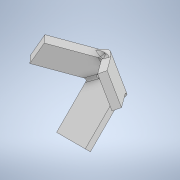
# Autodesk Inventor part: arm_holder_1
Saved by Autodesk Inventor 2020 (Build 240168000, 168)
## iProperties
Created: 2020-01-19
Part Number: arm_holder_1
Material: Generic
Document SubType Name: Modeling
Designer: psrobotics
Density: 1 g/cm^3
Appearance: Default
Author: psrobotics
Autodesk Inventor part; units mm, degrees
ref_plane "YZ Plane" through (0, 0, 0) normal (1, 0, 0) x (0, 1, 0)
ref_plane "XZ Plane" through (0, 0, 0) normal (0, 1, 0) x (-1, 0, 0)
ref_plane "XY Plane" through (0, 0, 0) normal (0, 0, 1) x (1, 0, 0)
sketch "Sketch1" plane through (0, 0, 0) normal (0, 0, 1) x (1, 0, 0)
  line L0 (0, 0) -> (20, 0)
  line L1 (20, 0) -> (10, 17.3205)
  line L2 (10, 17.3205) -> (0, 0)
  line L3 (10, 17.3205) -> (14.3301, 19.8205)
  line L4 (14.3301, 19.8205) -> (24.3301, 2.5)
  line L5 (24.3301, 2.5) -> (20, 0)
  line L6 (20, 0) -> (0, 0)
  line L7 (0, 0) -> (0, -5)
  line L8 (0, -5) -> (20, -5)
  line L9 (20, -5) -> (20, 0)
  line L10 (10, 17.3205) -> (5.6699, 19.8205)
  line L11 (5.6699, 19.8205) -> (-4.3301, 2.5)
  line L12 (-4.3301, 2.5) -> (0, 0)
  line L13 (5.6699, 19.8205) -> (14.3301, 19.8205)
  line L14 (20, -5) -> (24.3301, 2.5)
  line L15 (0, -5) -> (-4.3301, 2.5)
  dimension "d0" = 20
  dimension "d1" = 20
  dimension "d2" = 60
  dimension "d3" = 5
  dimension "d4" = 20
  dimension "d5" = 20
  dimension "d6" = 5
  dimension "d7" = 5
  dimension "d8" = 20
  dimension "d9" = 5
  constraints: 32 end point, 4 perpendicular, 2 horizontal, 2 parallel
  measures "d0" distance of L0.start L0.end
  measures "d1" distance of L0.end L1.end
  measures "d2" angle of L1 L0
  measures "d3" distance of L1.end L3.end
  measures "d4" distance of L3.end L4.end
  measures "d5" distance of L8.end L7.end
  measures "d6" distance of L7.end L6.end
  measures "d7" distance of L1.end L10.end
  measures "d8" distance of L10.end L11.end
  measures "d9" distance of L0.start L11.end
extrude "Extrusion1" add sketch "Sketch1" along normal blind 3 contours L12 L11 L10 L2 | L0 L9 L8 L7 | L7 L15 L12 | L1 L3 L4 L5 | L5 L14 L9 | L10 L13 L3
sketch "Sketch2" plane through (0, -5, 0) normal (0, -1, 0) x (1, 0, 0)
  line L0 (0, 0) -> (20, 0) projected
  line L1 (20, 0) -> (20, 3) projected
  line L2 (0, 3) -> (20, 3) projected
  line L3 (0, 0) -> (0, 3) projected
  line L4 (20, 3) -> (0, 3)
  line L5 (0, 3) -> (0, 23)
  line L6 (0, 23) -> (20, 23)
  line L7 (20, 23) -> (20, 3)
  dimension "d12" = 20
  dimension "d13" = 20
  constraints: 8 end point, 2 parallel, 1 horizontal, 1 perpendicular
  measures "d12" distance of L5.end L6.end
  measures "d13" distance of L4.end L5.end
extrude "Extrusion2" add sketch "Sketch2" along normal blind 20 contours L5 L6 L7 L2
sketch "Sketch3" plane through (0, -5, 3) normal (-1, 0, 0) x (0, 0, 1)
  line L0 (20, 0) -> (0, 0) projected
  line L1 (0, 0) -> (0, -20) projected
  line L2 (20, -20) -> (0, -20) projected
  line L3 (20, 0) -> (20, -20) projected
  line L4 (0, 0) -> (0, 7.5) projected
  line L5 (0, -20) -> (20, -20) projected
  line L6 (0, 0) -> (20, -20)
  point P0 (-3, 5)
  constraints: 2 end point
extrude "Extrusion3" cut sketch "Sketch3" against normal blind 20 contours L6 L2 L1
sketch "Sketch4" plane through (0, -5, 3) normal (-1, 0, 0) x (0, 0, 1)
  line L0 (0, 0) -> (20, -20) projected
  line L1 (20, 0) -> (20, -20) projected
  line L2 (20, 0) -> (0, 0) projected
  line L3 (0, 7.5) -> (0, 0) projected
  line L4 (20, -20) -> (23.5355, -16.4645)
  line L5 (0, 0) -> (20, -20) projected
  line L6 (23.5355, -16.4645) -> (-1.2132, 8.2843)
  line L7 (-3, 0) -> (0, 0) projected
  line L8 (0, 0) -> (0, 7.0711)
  point P0 (-3, 5)
  point P1 (7.0711, 0)
  point P2 (20, -12.9289)
  dimension "d18" = 5
  dimension "d19" = 35
  constraints: 6 end point, 2 perpendicular, 2 point on line
  measures "d18" distance of L0.end L4.end
  measures "d19" distance of L4.end L6.end
extrude "Extrusion4" cut sketch "Sketch4" against normal blind 20 contours L2 L1 L6
sketch "Sketch5" plane through (0, -5, 3) normal (-1, 0, 0) x (0, 0, 1)
  line L0 (20, -12.9289) -> (7.0711, 0) projected
  line L1 (7.0711, 0) -> (0, 0) projected
  line L2 (0, 0) -> (20, -20) projected
  line L3 (20, -12.9289) -> (20, -20) projected
  line L4 (7.0711, 0) -> (0, 0) projected
  line L5 (7.0711, 0) -> (0, 7.0711)
  line L6 (0, 0) -> (0, 7.5) projected
  line L7 (0, 7.0711) -> (0, 0)
  line L8 (0, 22.3205) -> (0, 5) projected
  point P0 (-3, 5)
  constraints: 4 end point, 2 collinear, 1 point on line
extrude "Extrusion5" add sketch "Sketch5" against normal up to surface (20 mm away) contours L1 L6 L5
sketch "Sketch6" plane through (20, 0, 3) normal (0, 0, -1) x (-1, 0, 0)
  line L0 (1.1957, 2.0711) -> (0, 0) projected
  line L1 (0, 0) -> (20, 0) projected
  line L2 (20, 0) -> (18.8043, 2.0711) projected
  line L3 (18.8043, 2.0711) -> (1.1957, 2.0711) projected
  point P0 (20, 0)
extrude "Extrusion6" add sketch "Sketch6" along normal up to surface (3 mm away)
sketch "Sketch7" plane through (0, 0, 3) normal (0, 0, 1) x (1, 0, 0)
  line L0 (0, -5) -> (20, -5) projected
  line L1 (24.3301, 2.5) -> (14.3301, 19.8205) projected
  line L2 (5.6699, 19.8205) -> (-4.3301, 2.5) projected
  line L3 (0.6699, 11.1603) -> (10, 5.7735)
  line L4 (10, 5.7735) -> (19.3301, 11.1603)
  line L5 (10, 5.7735) -> (10, -5)
  line L6 (0, -5) -> (20, -5) projected
  line L7 (5.6699, 19.8205) -> (-4.3301, 2.5) projected
  line L8 (24.3301, 2.5) -> (14.3301, 19.8205) projected
  circle A0 centre (10, 5.7735) radius 1.5
  point P0 (0, 0)
  dimension "d26" = 3
  constraints: 6 end point, 3 midpoint, 3 perpendicular, 1 centre point, 1 coincident
  measures "d26" diameter of A0
extrude "Extrusion7" add sketch "Sketch7" along normal blind 5
pattern_circular "Circular Pattern1" count 3 over 360 about axis through (10, 5.7735, 3) along (0, 0, 1) of "Extrusion2", "Extrusion3", "Extrusion4", "Extrusion5", "Extrusion6"
sketch "Sketch8" plane through (10, 5.7735, 8) normal (0, 0, 1) x (1, 0, 0)
  circle A0 centre (0, 0) radius 1.5 projected
  point P0 (-10, -5.7735)
extrude "Extrusion8" cut sketch "Sketch8" against normal blind 5
fillet "Fillet1" radius 1 3 edges at (16.4128, 2.0711, 1.5) (10, 13.1784, 1.5) (3.5872, 2.0711, 1.5)
fillet "Fillet2" radius 2 6 edges at (2.2266, 1.2855, 3.7855) (10, 14.7494, 3.7855) (17.7734, 1.2855, 3.7855) (20, 0, 4.0355) (10, 17.3205, 4.0355) (0, 0, 4.0355)
fillet "Fillet3" radius 2 9 edges at (-0.2679, -0.1547, 3) (0, -3.0774, 3) (-2.6651, 1.5387, 3) (10, 17.6299, 3) (7.3349, 18.8592, 3) (12.6651, 18.8592, 3) (20, -3.0774, 3) (22.6651, 1.5387, 3) (20.2679, -0.1547, 3)
chamfer "Chamfer1" distance 3 angle 45 3 edges at (10, -5, 0) (19.3301, 11.1603, 0) (0.6699, 11.1603, 0)
sketch "Sketch9" plane through (20, -25, 23) normal (1, 0, 0) x (0, 0, -1)
  line L0 (18, 23.8453) -> (18, 20) projected
  line L1 (16.7483, 23.8453) -> (18, 23.8453) projected
  ellipse E0 centre (15.1005, 25) end of major axis (16.9262, 26.8257) minor radius 2 (16.5147, 23.5858) -> (16.7483, 23.8453) ccw projected
  line L2 (0, 7.0711) -> (16.5147, 23.5858) projected
  line L3 (0, 7.0711) -> (0, 0) projected
  line L4 (0, 0) -> (20, 20) projected
  line L5 (20, 20) -> (18, 20) projected
  line L6 (0, 7.0711) -> (16.5147, 23.5858) projected
  line L7 (0, 7.0711) -> (-3.5355, 3.5355)
  line L8 (-3.5355, 3.5355) -> (0, 0)
  line L9 (0, 0) -> (20, 20) projected
  point P0 (23, 25)
  constraints: 4 end point, 1 parallel, 1 perpendicular, 1 other
extrude "Extrusion9" add sketch "Sketch9" against normal up to surface (20 mm away) contours L8 L7 L3
sketch "Sketch10" plane through (5.6699, 19.8205, 5) normal (0.5, 0.8660254, 0) x (0.8660254, -0.5, 0)
  line L0 (0, 0) -> (3.8453, 0) projected
  line L1 (0, 0) -> (0, 2) projected
  line L2 (0, 2) -> (-20, -18) projected
  line L3 (-12.9289, -18) -> (-20, -18) projected
  line L4 (-12.9289, -18) -> (3.5858, -1.4853) projected
  ellipse E0 centre (5, -2.8995) end of major axis (6.8257, -1.0738) minor radius 2 (3.8453, -1.2517) -> (3.5858, -1.4853) ccw projected
  line L5 (3.8453, 0) -> (3.8453, -1.2517) projected
  line L6 (-12.9289, -18) -> (-16.4645, -21.5355)
  line L7 (-16.4645, -21.5355) -> (-20, -18)
  point P0 (5, 5)
  constraints: 4 end point, 1 perpendicular, 1 point on line, 1 other
extrude "Extrusion10" add sketch "Sketch10" against normal up to surface (20 mm away) contours L3 L6 L7
sketch "Sketch11" plane through (24.3301, 2.5, 3) normal (0.5, -0.8660254, 0) x (0.8660254, 0.5, 0)
  line L0 (0, 2) -> (-3.8453, 2) projected
  line L1 (0, 2) -> (0, 0) projected
  line L2 (0, 0) -> (20, 20) projected
  line L3 (12.9289, 20) -> (20, 20) projected
  line L4 (12.9289, 20) -> (-3.5858, 3.4853) projected
  ellipse E0 centre (-5, 4.8995) end of major axis (-6.8257, 3.0738) minor radius 2 (-3.8453, 3.2517) -> (-3.5858, 3.4853) ccw projected
  line L5 (-3.8453, 2) -> (-3.8453, 3.2517) projected
  line L6 (12.9289, 20) -> (20, 20) projected
  line L7 (12.9289, 20) -> (16.4645, 23.5355)
  line L8 (16.4645, 23.5355) -> (20, 20)
  point P0 (-22.3205, -3)
  constraints: 4 end point, 1 parallel, 1 perpendicular, 1 other
extrude "Extrusion11" add sketch "Sketch11" against normal up to surface (20 mm away) contours L3 L7 L8
body "Solid1"
